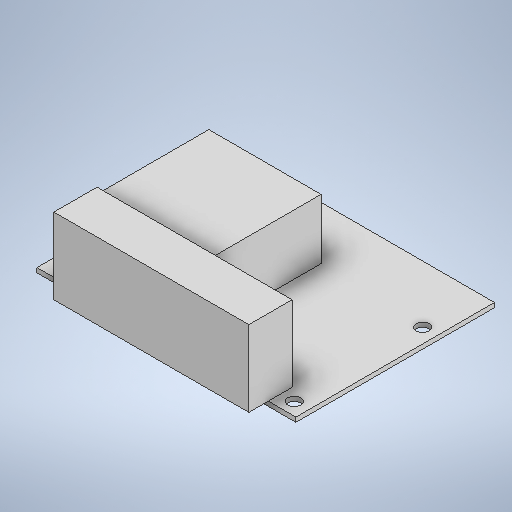
# Autodesk Inventor part: CapCharger
Saved by Autodesk Inventor 2025.1 (Build 291241000, 241)
## iProperties
Created: 2025-05-21
Part Number: CapCharger
Material: Generic
Document SubType Name: Modeling
Designer: User
Density: 1 g/cm^3
Appearance: Default
Author: User
Autodesk Inventor part; units mm, degrees
ref_plane "YZ Plane" through (0, 0, 0) normal (1, 0, 0) x (0, 1, 0)
ref_plane "XZ Plane" through (0, 0, 0) normal (0, 1, 0) x (-1, 0, 0)
ref_plane "XY Plane" through (0, 0, 0) normal (0, 0, 1) x (1, 0, 0)
sketch "Sketch1" plane through (0, 0, 0) normal (0, 1, 0) x (-1, 0, 0)
  line L0 (8.4436, 19.7296) -> (-51.5564, 19.7296)
  line L1 (-51.5564, 19.7296) -> (-51.5564, -26.2704)
  line L2 (-51.5564, -26.2704) -> (8.4436, -26.2704)
  line L3 (8.4436, -26.2704) -> (8.4436, 19.7296)
  point P0 (0, 0)
  dimension "d0" = 60
  dimension "d1" = 46
  constraints: 8 end point, 2 parallel, 1 horizontal, 1 perpendicular
  measures "d0" distance of L2.end L1.end
  measures "d1" distance of L1.end L0.end
extrude "Extrusion1" add sketch "Sketch1" along normal blind 3.7
sketch "Sketch2" plane through (0, 3.7, 0) normal (0, 1, 0) x (1, 0, 0)
  line L0 (-8.4436, -19.7296) -> (51.5564, -19.7296) projected
  line L1 (-8.4436, 26.2704) -> (-8.4436, -19.7296) projected
  line L2 (51.5564, -19.7296) -> (51.5564, 26.2704) projected
  line L3 (-8.4436, -19.7296) -> (-0.0236, -19.7296)
  line L4 (51.5564, -19.7296) -> (45.1564, -19.7296)
  line L5 (45.1564, -19.7296) -> (45.1564, -14.2296)
  line L6 (45.1564, -14.2296) -> (-0.0236, -14.2296)
  line L7 (-0.0236, -14.2296) -> (-0.0236, -24.2296)
  line L8 (-0.0236, -24.2296) -> (45.1564, -24.2296)
  line L9 (45.1564, -24.2296) -> (45.1564, -14.2296)
  point P0 (0, 0)
  dimension "d4" = 8.42
  dimension "d5" = 6.4
  dimension "d6" = 5.5
  dimension "d7" = 10
  constraints: 14 end point, 2 parallel, 2 point on line, 1 horizontal, 1 perpendicular, 1 vertical
  measures "d4" distance of L0.start L3.end
  measures "d5" distance of L0.end L4.end
  measures "d6" distance of L4.end L5.end
  measures "d7" distance of L7.end L6.end
extrude "Extrusion2" add sketch "Sketch2" along normal blind 17.6
sketch "Sketch3" plane through (0, 3.7, 0) normal (0, 1, 0) x (1, 0, 0)
  line L0 (-8.4436, 26.2704) -> (-8.4436, -19.7296) projected
  line L1 (-2.3236, 26.2704) -> (-2.3236, -19.7296)
  line L2 (45.1564, -14.2296) -> (-0.0236, -14.2296) projected
  line L3 (45.1564, -12.5296) -> (-0.0236, -12.5296)
  line L4 (-2.3236, -12.5296) -> (23.6764, -12.5296)
  line L5 (23.6764, -12.5296) -> (23.6764, 13.9704)
  line L6 (23.6764, 13.9704) -> (-2.3236, 13.9704)
  line L7 (-2.3236, 13.9704) -> (-2.3236, -12.5296)
  point P0 (0, 0)
  dimension "d10" = 6.12
  dimension "d11" = 1.7
  dimension "d12" = 26
  dimension "d13" = 26.5
  constraints: 12 end point, 4 parallel, 1 horizontal, 1 perpendicular, 1 point on line
  measures "d10" distance between parallel lines of L0 L1
  measures "d11" distance between parallel lines of L2 L3
  measures "d12" distance of L6.end L5.end
  measures "d13" distance of L5.end L4.end
extrude "Extrusion3" add sketch "Sketch3" along normal blind 13.9
sketch "Sketch4" plane through (0, 3.7, 0) normal (0, 1, 0) x (1, 0, 0)
  line L0 (-8.4436, -19.7296) -> (-0.0236, -19.7296) projected
  line L1 (-6.5036, 26.2704) -> (-6.5036, -17.7896)
  line L2 (-0.0236, -18.3496) -> (-7.0636, -18.3496)
  circle A0 centre (-5.0036, -16.8496) radius 1.5
  line L3 (51.5564, 26.2704) -> (-8.4436, 26.2704) projected
  line L4 (51.5564, 24.8704) -> (-7.0436, 24.8704)
  circle A1 centre (-5.0036, 23.3704) radius 1.5
  line L5 (49.7164, -19.7296) -> (49.7164, 24.4304)
  line L6 (-0.0236, -41.0522) -> (-29.7662, -41.0522)
  line L7 (-29.7662, -41.0522) -> (-29.7662, 47.593)
  line L8 (-29.7662, 47.593) -> (72.879, 47.593)
  line L9 (72.879, 47.593) -> (72.879, -19.7296)
  line L10 (45.1564, -19.7296) -> (51.5564, -19.7296) projected
  line L11 (45.1564, -18.2796) -> (50.1064, -18.2796)
  circle A2 centre (48.2164, -16.7796) radius 1.5
  line L12 (51.5564, 14.4704) -> (-7.0436, 14.4704)
  circle A3 centre (48.2164, 12.9704) radius 1.5
  point P0 (0, 0)
  dimension "d17" = 1.38
  dimension "d18" = 3
  dimension "d19" = 1.4
  dimension "d20" = 3
  dimension "d22" = 1.45
  dimension "d23" = 3
  dimension "d24" = 10.4
  dimension "d25" = 3
  constraints: 20 end point, 8 tangent, 4 centre point, 1 parallel
  measures "d17" distance between parallel lines of L0 L2
  measures "d18" diameter of A0
  measures "d19" distance between parallel lines of L3 L4
  measures "d20" diameter of A1
  measures "d22" distance between parallel lines of L10 L11
  measures "d23" diameter of A2
  measures "d24" distance between parallel lines of L4 L12
  measures "d25" diameter of A3
extrude "Extrusion4" cut sketch "Sketch4" against normal blind 13.9 contours A1 | A0 | A2 | A3
sketch "Sketch5" plane through (0, 0, 0) normal (0, -1, 0) x (1, 0, 0)
  line L0 (51.5564, 19.7296) -> (51.5564, -26.2704) projected
  line L1 (-8.4436, 19.7296) -> (51.5564, 19.7296) projected
  line L2 (-8.4436, -26.2704) -> (-8.4436, 19.7296) projected
  line L3 (51.5564, -26.2704) -> (-8.4436, -26.2704) projected
  line L4 (43.9969, -18.7109) -> (43.9969, 12.1701)
  line L5 (43.9969, 12.1701) -> (-0.8841, 12.1701)
  line L6 (-0.8841, 12.1701) -> (-0.8841, -18.7109)
  line L7 (-0.8841, -18.7109) -> (43.9969, -18.7109)
  point P0 (0, 0)
  constraints: 8 end point, 3 other
extrude "Extrusion5" cut sketch "Sketch5" against normal blind 2.65
body "Solid1"
